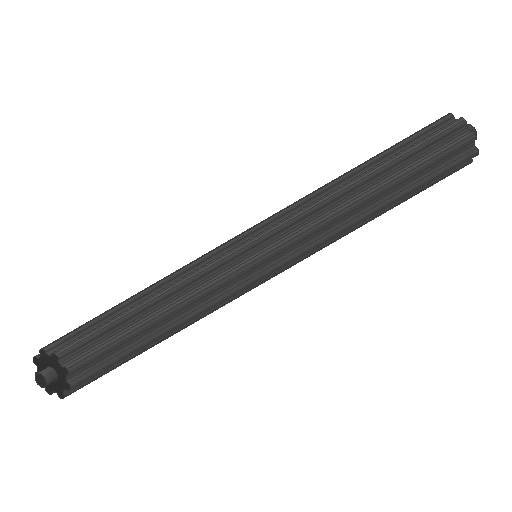
# Autodesk Inventor part: Coletor - Intake
Saved by Autodesk Inventor 2027.1 (Build 311270010, 270A)
## iProperties
Created: 2026-05-13
Part Number: Coletor - Intake
Material: Genérico
Document SubType Name: Modeling
Designer: djair.oliveira
Density: 1 g/cm^3
Appearance: Padrão
Author: djair.oliveira
Autodesk Inventor part; units mm, degrees
ref_plane "YZ Plane" through (0, 0, 0) normal (1, 0, 0) x (0, 1, 0)
ref_plane "XZ Plane" through (0, 0, 0) normal (0, 1, 0) x (-1, 0, 0)
ref_plane "XY Plane" through (0, 0, 0) normal (0, 0, 1) x (1, 0, 0)
sketch "Esboço1" plane through (0, 0, 0) normal (1, 0, 0) x (0, 1, 0)
  line L0 (0, 0) -> (0, -572.55)
  line L1 (0, 0) -> (7.5, 0)
  line L2 (7.5, 0) -> (7.5, -572.55)
  line L3 (7.5, -572.55) -> (0, -572.55)
  line L4 (0, -572.55) -> (0, 0)
  line L5 (7.5, -15) -> (25.4, -15)
  line L6 (25.4, -15) -> (25.4, -557.55)
  line L7 (25.4, -557.55) -> (7.5, -557.55)
  line L8 (7.5, -557.55) -> (7.5, -15)
  point P0 (3.75, 0)
  point P1 (3.75, -572.55)
  point P2 (0, -545.49)
  point P3 (7.5, -557.55)
  dimension "d0" = 572.55
  dimension "d1" = 7.5
  dimension "d2" = 25.4
  dimension "d3" = 15
  dimension "d4" = 15
  constraints: 18 end point, 4 parallel, 2 horizontal, 2 midpoint, 2 perpendicular, 2 point on line, 1 vertical
  measures "d0" distance of L0.start L0.end
  measures "d1" distance of L2.end L3.end
  measures "d2" distance between parallel lines of L0 L6
  measures "d3" distance from line of point (3.75, 0) L5
  measures "d4" distance from line of point (3.75, -572.55) L7
revolve "Revolução1" add sketch "Esboço1" angle 360 about axis through (0, 0, -572.55) along (0, 0, 1)
sketch "Esboço2" plane through (0, 0, -15) normal (0, 0, 1) x (1, 0, 0)
  circle A0 centre (0, 0) radius 7.5 projected
  circle A1 centre (0, 0) radius 25.4 projected
  circle A2 centre (0, 0) radius 7.5 projected
  line L0 (0, 0) -> (0, 25.4)
  line L1 (0, 0) -> (-25.4, 0)
  line L2 (0, 0) -> (0, -25.4)
  line L3 (0, 0) -> (25.4, 0)
  line L4 (0, 0) -> (17.9605, 17.9605)
  line L5 (0, 0) -> (9.7202, 23.4665)
  line L6 (0, 0) -> (23.4665, 9.7202)
  line L7 (0, 0) -> (-17.9605, 17.9605)
  line L8 (0, 0) -> (-9.7202, 23.4665)
  line L9 (0, 0) -> (-23.4665, 9.7202)
  line L10 (0, 0) -> (17.9605, -17.9605)
  line L11 (0, 0) -> (9.7202, -23.4665)
  line L12 (0, 0) -> (23.4665, -9.7202)
  line L13 (0, 0) -> (-9.7202, -23.4665)
  line L14 (0, 0) -> (-17.9605, -17.9605)
  line L15 (0, 0) -> (-23.4665, -9.7202)
  circle A3 centre (0, 0) radius 19.4
  point P0 (0, 0)
  point P1 (-17.9233, 7.4241)
  point P2 (-13.7179, 13.7179)
  point P3 (-17.9233, -7.4241)
  point P4 (-19.4, 0)
  point P5 (-7.4241, -17.9233)
  point P6 (-13.7179, -13.7179)
  point P7 (7.4241, -17.9233)
  point P8 (0, -19.4)
  point P9 (17.9233, -7.4241)
  point P10 (13.7179, -13.7179)
  point P11 (17.9233, 7.4241)
  point P12 (19.4, 0)
  point P13 (7.4241, 17.9233)
  point P14 (13.7179, 13.7179)
  point P15 (-7.4241, 17.9233)
  point P16 (0, 19.4)
  dimension "d8" = 22.5
  dimension "d9" = 22.5
  dimension "d10" = 45
  dimension "d11" = 6
  constraints: 32 end point, 9 symmetric about line, 2 point on line, 1 centre point, 1 coincident, 1 perpendicular, 1 vertical, 8 other
  measures "d8" angle of L3 L6
  measures "d9" angle of L0 L5
  measures "d10" angle of L3 L4
extrude "Extrusão1" cut sketch "Esboço2" against normal up to surface (542.55 mm away) contours A3 L6 A1 L3 | L12 A1 L10 A3 | A3 L5 A1 L4 | A3 L8 A1 L0 | A3 L15 A1 L1 | A3 L11 A1 L2 | A3 L9 A1 L7 | L13 A1 L14 A3
fillet "Arredondamento1" radius 3 31 edges at (7.4241, 17.9233, -286.275) (13.7179, 13.7179, -286.275) (17.9605, 17.9605, -286.275) (9.7202, 23.4665, -286.275) (0, 25.4, -286.275) (0, 19.4, -286.275) (-9.7202, 23.4665, -286.275) (-7.4241, 17.9233, -286.275) (-23.4665, 9.7202, -286.275) (-17.9605, 17.9605, -286.275) (-17.9233, 7.4241, -286.275) (-13.7179, 13.7179, -286.275) (19.4, 0, -286.275) (17.9233, 7.4241, -286.275) (23.4665, 9.7202, -286.275) (25.4, 0, -286.275) (23.4665, -9.7202, -286.275) (17.9233, -7.4241, -286.275) (17.9605, -17.9605, -286.275) (13.7179, -13.7179, -286.275) (7.4241, -17.9233, -286.275) (9.7202, -23.4665, -286.275) (0, -19.4, -286.275) (-9.7202, -23.4665, -286.275) (-7.4241, -17.9233, -286.275) (-13.7179, -13.7179, -286.275) (-23.4665, -9.7202, -286.275) (-17.9605, -17.9605, -286.275) (-19.4, 0, -286.275) (-25.4, 0, -286.275) (0, -25.4, -286.275)
equation "\"d9\" = d8"
